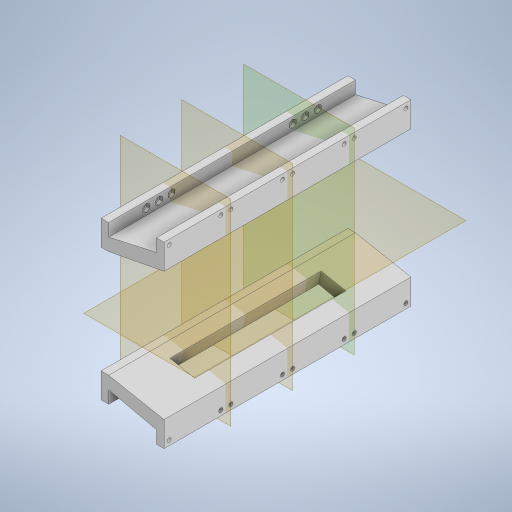
# Autodesk Inventor part: Antenna holder
Saved by Autodesk Inventor 2023.5 (Build 275446000, 446)
## iProperties
Created: 2025-10-16
Part Number: Antenna holder
Material: Generic
Document SubType Name: Modeling
Designer: Mikke
Density: 1 g/cm^3
Appearance: Default
Author: Mikke
Autodesk Inventor part; units mm, degrees
ref_plane "YZ Plane" through (0, 0, 0) normal (1, 0, 0) x (0, 1, 0)
ref_plane "XZ Plane" through (0, 0, 0) normal (0, 1, 0) x (-1, 0, 0)
ref_plane "XY Plane" through (0, 0, 0) normal (0, 0, 1) x (1, 0, 0)
sketch "Sketch4" plane through (0, 0, 0) normal (0, 0, 1) x (1, 0, 0)
  line L0 (-0.75, -71) -> (0.75, -71)
  line L1 (0.75, -71) -> (0.75, 71)
  line L2 (0.75, 71) -> (-0.75, 71)
  line L3 (-0.75, 71) -> (-0.75, -71)
  line L4 (-0.75, -71) -> (0.75, 71) construction
  line L5 (0.75, -71) -> (-0.75, 71) construction
  line L6 (-0.75, 71) -> (-6.75, 71)
  line L7 (-6.75, 71) -> (-6.75, 51)
  line L8 (-6.75, 51) -> (-0.75, 51)
  line L9 (-0.75, 51) -> (-0.75, 71)
  line L10 (-0.75, -71) -> (-6.75, -71)
  line L11 (-6.75, -71) -> (-6.75, -51)
  line L12 (-6.75, -51) -> (-0.75, -51)
  line L13 (-0.75, -51) -> (-0.75, -71)
  line L14 (-0.75, 0) -> (-50.75, 0)
  line L15 (-0.75, 0) -> (49.25, 0) construction
  line L16 (-0.75, 0) -> (-3.75, 0)
  line L17 (-6.75, -3) -> (-0.75, -3)
  line L18 (-0.75, -3) -> (-0.75, 3)
  line L19 (-0.75, 3) -> (-6.75, 3)
  line L20 (-6.75, 3) -> (-6.75, -3)
  line L21 (-6.75, -3) -> (-0.75, 3) construction
  line L22 (-0.75, -3) -> (-6.75, 3) construction
  line L23 (-6.75, 51) -> (-6.75, 61)
  line L24 (-6.75, -51) -> (-6.75, -61)
  line L25 (-50.75, 0) -> (-50.75, 62.5)
  line L26 (-50.75, 0) -> (-50.75, -62.5)
  line L27 (-50.75, 62.5) -> (-50.75, 52.5)
  line L28 (-50.75, -62.5) -> (-50.75, -62.5)
  line L29 (-50.75, 62.5) -> (-50.75, 57.5)
  line L30 (-50.75, -52.5) -> (-50.75, -57.5)
  line L31 (-50.75, 62.5) -> (-50.75, 42.5)
  line L32 (-50.75, 42.5) -> (-44.75, 42.5)
  line L33 (-44.75, 42.5) -> (-44.75, 62.5)
  line L34 (-44.75, 62.5) -> (-50.75, 62.5)
  line L35 (-50.75, 52.5) -> (-44.75, 52.5)
  line L36 (-44.75, 52.5) -> (-6.75, 61)
  line L37 (-50.75, -62.5) -> (-50.75, -42.5)
  line L38 (-50.75, -42.5) -> (-44.75, -42.5)
  line L39 (-44.75, -42.5) -> (-44.75, -62.5)
  line L40 (-44.75, -62.5) -> (-50.75, -62.5)
  line L41 (-50.75, -52.5) -> (-44.75, -52.5)
  line L42 (-44.75, -52.5) -> (-6.75, -61)
  line L43 (-44.75, -42.5) -> (-0.75, -51)
  line L44 (-44.75, 42.5) -> (-0.75, 51)
  point P0 (0, 0)
  point P1 (-0.75, -51)
  dimension "d22" = 1.5
  dimension "d23" = 142
  dimension "d24" = 6
  dimension "d25" = 20
  dimension "d26" = 6
  dimension "d27" = 20
  dimension "d28" = 50
  dimension "d29" = 180
  dimension "d36" = 6
  dimension "d37" = 6
  dimension "d38" = 10
  dimension "d39" = 10
  dimension "d45" = 62.5
  dimension "d46" = 62.5
  dimension "d47" = 10
  dimension "d55" = 115
  dimension "d56" = 20
  dimension "d57" = 6
  dimension "d58" = 20
  dimension "d59" = 6
  dimension "d60" = 20
  constraints: 90 end point, 10 midpoint, 9 perpendicular, 8 parallel, 6 horizontal, 5 point on line, 1 collinear, 1 vertical
  measures "d22" distance of L2.end L1.end
  measures "d23" distance of L1.end L0.end
  measures "d24" distance of L8.end L7.end
  measures "d25" distance of L7.end L6.end
  measures "d26" distance of L11.end L12.end
  measures "d27" distance of L10.end L11.end
  measures "d28" distance of L14.start L14.end
  measures "d29" angle of L14 L15
  measures "d36" distance of L19.end L18.end
  measures "d37" distance of L18.end L17.end
  measures "d38" distance of L7.end L23.end
  measures "d39" distance of L11.end L24.end
  measures "d45" distance of L14.end L25.end
  measures "d46" distance of L14.end L26.end
  measures "d47" distance of L25.end L27.end
  measures "d55" distance of L30.end L29.end
  measures "d56" distance of L25.end L31.end
  measures "d57" distance of L31.end L32.end
  measures "d58" distance of L28.start L37.end
  measures "d59" distance of L37.end L38.end
  measures "d60" distance of L38.end L39.end
extrude "Extrusion3" add sketch "Sketch4" along normal mid plane 196 contours L10 L11 L12 L3 | L12 L11 L42 L39 L43 | L39 L41 L26 L38 | L3 L8 L7 L6 | L39 L40 L26 L41 | L44 L33 L36 L7 L8 | L32 L25 L35 L33 | L35 L25 L34 L33
ref_plane "Work Plane4" through (0, 0, 0) normal (0, 0, 1) x (1, 0, 0)
ref_plane "Work Plane5" through (0, 0, -49) normal (0, 0, -1) x (-1, 0, 0)
ref_plane "Work Plane6" through (0, 0, 49) normal (0, 0, 1) x (1, 0, 0)
ref_plane "Work Plane7" through (-50.75, 0, 98) normal (0, 1, 0) x (1, 0, 0)
sketch "Sketch9" plane through (-6.75, 61, 98) normal (-1, 0, 0) x (0, 0, 1)
  line L0 (0, 10) -> (0, 0) projected
  line L1 (0, 10) -> (-24.5, 10)
  line L2 (0, 10) -> (-196, 10) projected
  line L3 (-24.5, 10) -> (-4, 10)
  line L4 (-24.5, 10) -> (-45, 10)
  line L5 (-45, 10) -> (-45, 6)
  line L6 (-45, 6) -> (-42.25, 6)
  line L7 (-4, 10) -> (-4, 6)
  line L8 (-4, 6) -> (-6.75, 6)
  line L9 (-6.75, 7.5877) -> (-4, 9.1754)
  line L10 (-4, 9.1754) -> (-1.25, 7.5877)
  line L11 (-1.25, 7.5877) -> (-1.25, 4.4123)
  line L12 (-1.25, 4.4123) -> (-4, 2.8246)
  line L13 (-4, 2.8246) -> (-6.75, 4.4123)
  line L14 (-6.75, 4.4123) -> (-6.75, 7.5877)
  line L15 (-42.25, 4.4123) -> (-45, 2.8246)
  line L16 (-45, 2.8246) -> (-47.75, 4.4123)
  line L17 (-47.75, 4.4123) -> (-47.75, 7.5877)
  line L18 (-47.75, 7.5877) -> (-45, 9.1754)
  line L19 (-45, 9.1754) -> (-42.25, 7.5877)
  line L20 (-42.25, 7.5877) -> (-42.25, 4.4123)
  point P0 (-98, -61)
  dimension "d88" = 24.5
  dimension "d89" = 20.5
  dimension "d90" = 20.5
  dimension "d91" = 4
  dimension "d92" = 2.75
  dimension "d93" = 4
  dimension "d94" = 2.75
  constraints: 38 end point, 3 point on line, 2 coincident, 2 horizontal, 2 midpoint, 2 perpendicular, 26 other
  measures "d88" distance of L0.start L1.end
  measures "d89" distance of L1.end L3.end
  measures "d90" distance of L1.end L4.end
  measures "d91" distance of L4.end L5.end
  measures "d92" distance of L5.end L6.end
  measures "d93" distance of L3.end L7.end
  measures "d94" distance of L7.end L8.end
extrude "Extrusion7" cut sketch "Sketch9" against normal blind 2.5
sketch "Sketch10" plane through (-4.25, 61, 98) normal (-1, 0, 0) x (0, 0, 1)
  line L0 (-4, 2.8246) -> (-6.75, 4.4123) projected
  line L1 (-4, 2.8246) -> (-4, 6.0001)
  circle A0 centre (-4, 6.0001) radius 1.55
  line L2 (-42.25, 4.4123) -> (-45, 2.8246) projected
  line L3 (-45, 2.8246) -> (-45, 6.0001)
  circle A1 centre (-45, 6.0001) radius 1.55
  point P0 (-98, -61)
  dimension "d97" = 3.1755
  dimension "d98" = 3.1
  dimension "d99" = 3.1755
  dimension "d100" = 3.1
  constraints: 4 end point, 2 centre point, 2 coincident, 2 vertical
  measures "d97" distance of L0.start L1.end
  measures "d98" diameter of A0
  measures "d99" distance of L2.end L3.end
  measures "d100" diameter of A1
extrude "Extrusion8" cut sketch "Sketch10" against normal blind 6
mirror "Mirror4" about plane through (0, 0, 49) normal (0, 0, 1) of "Extrusion7", "Extrusion8"
mirror "Mirror5" about plane through (0, 0, 0) normal (0, 0, 1) of "Extrusion7", "Extrusion8", "Mirror4"
mirror "Mirror6" about plane through (-50.75, 0, 98) normal (0, 1, 0) of "Extrusion7", "Extrusion8", "Mirror4", "Mirror5"
sketch "Sketch11" plane through (-44.75, 52.5, 98) normal (1, 0, 0) x (0, 0, -1)
  line L0 (196, 10) -> (0, 10) projected
  line L1 (98, 10) -> (49.925, 10)
  line L2 (196, 10) -> (0, 10) projected
  line L3 (98, 10) -> (146.075, 10)
  line L4 (49.925, 10) -> (49.925, 5)
  line L5 (49.925, 5) -> (52.675, 5)
  line L6 (146.075, 10) -> (146.075, 5)
  line L7 (146.075, 5) -> (143.325, 5)
  line L8 (49.925, 5) -> (39.925, 5)
  line L9 (39.925, 5) -> (42.675, 5)
  line L10 (39.925, 5) -> (29.925, 5)
  line L11 (29.925, 5) -> (32.675, 5)
  line L12 (146.075, 5) -> (156.075, 5)
  line L13 (156.075, 5) -> (153.325, 5)
  line L14 (156.075, 5) -> (166.075, 5)
  line L15 (166.075, 5) -> (163.325, 5)
  line L16 (143.325, 6.5877) -> (146.075, 8.1754)
  line L17 (146.075, 8.1754) -> (148.825, 6.5877)
  line L18 (148.825, 6.5877) -> (148.825, 3.4123)
  line L19 (148.825, 3.4123) -> (146.075, 1.8246)
  line L20 (146.075, 1.8246) -> (143.325, 3.4123)
  line L21 (143.325, 3.4123) -> (143.325, 6.5877)
  line L22 (153.325, 6.5877) -> (156.075, 8.1754)
  line L23 (156.075, 8.1754) -> (158.825, 6.5877)
  line L24 (158.825, 6.5877) -> (158.825, 3.4123)
  line L25 (158.825, 3.4123) -> (156.075, 1.8246)
  line L26 (156.075, 1.8246) -> (153.325, 3.4123)
  line L27 (153.325, 3.4123) -> (153.325, 6.5877)
  line L28 (163.325, 6.5877) -> (166.075, 8.1754)
  line L29 (166.075, 8.1754) -> (168.825, 6.5877)
  line L30 (168.825, 6.5877) -> (168.825, 3.4123)
  line L31 (168.825, 3.4123) -> (166.075, 1.8246)
  line L32 (166.075, 1.8246) -> (163.325, 3.4123)
  line L33 (163.325, 3.4123) -> (163.325, 6.5877)
  line L34 (52.675, 3.4123) -> (49.925, 1.8246)
  line L35 (49.925, 1.8246) -> (47.175, 3.4123)
  line L36 (47.175, 3.4123) -> (47.175, 6.5877)
  line L37 (47.175, 6.5877) -> (49.925, 8.1754)
  line L38 (49.925, 8.1754) -> (52.675, 6.5877)
  line L39 (52.675, 6.5877) -> (52.675, 3.4123)
  line L40 (42.675, 3.4123) -> (39.925, 1.8246)
  line L41 (39.925, 1.8246) -> (37.175, 3.4123)
  line L42 (37.175, 3.4123) -> (37.175, 6.5877)
  line L43 (37.175, 6.5877) -> (39.925, 8.1754)
  line L44 (39.925, 8.1754) -> (42.675, 6.5877)
  line L45 (42.675, 6.5877) -> (42.675, 3.4123)
  line L46 (32.675, 3.4123) -> (29.925, 1.8246)
  line L47 (29.925, 1.8246) -> (27.175, 3.4123)
  line L48 (27.175, 3.4123) -> (27.175, 6.5877)
  line L49 (27.175, 6.5877) -> (29.925, 8.1754)
  line L50 (29.925, 8.1754) -> (32.675, 6.5877)
  line L51 (32.675, 6.5877) -> (32.675, 3.4123)
  point P0 (98, -52.5)
  point P1 (98, -52.5)
  dimension "d103" = 48.075
  dimension "d104" = 48.075
  dimension "d105" = 5
  dimension "d106" = 2.75
  dimension "d107" = 5
  dimension "d108" = 2.75
  dimension "d109" = 10
  dimension "d110" = 2.75
  dimension "d111" = 10
  dimension "d112" = 2.75
  dimension "d113" = 10
  dimension "d114" = 2.75
  dimension "d115" = 10
  dimension "d116" = 2.75
  constraints: 100 end point, 7 coincident, 7 midpoint, 6 point on line, 4 horizontal, 3 perpendicular, 1 vertical, 78 other
  measures "d103" distance of L1.start L1.end
  measures "d104" distance of L1.start L3.end
  measures "d105" distance of L1.end L4.end
  measures "d106" distance of L4.end L5.end
  measures "d107" distance of L3.end L6.end
  measures "d108" distance of L6.end L7.end
  measures "d109" distance of L4.end L8.end
  measures "d110" distance of L8.end L9.end
  measures "d111" distance of L8.end L10.end
  measures "d112" distance of L10.end L11.end
  measures "d113" distance of L6.end L12.end
  measures "d114" distance of L12.end L13.end
  measures "d115" distance of L12.end L14.end
  measures "d116" distance of L14.end L15.end
extrude "Extrusion9" cut sketch "Sketch11" against normal blind 2.5
sketch "Sketch12" plane through (-47.25, 52.5, 98) normal (1, 0, 0) x (0, 0, -1)
  line L0 (166.075, 1.8246) -> (166.075, 5.0001)
  line L1 (166.075, 5.0001) -> (156.0758, 4.8772)
  line L2 (156.0758, 4.8772) -> (146.0765, 4.7544)
  circle A0 centre (146.0765, 4.7544) radius 1.55
  circle A1 centre (156.0758, 4.8772) radius 1.55
  circle A2 centre (166.075, 5.0001) radius 1.55
  line L3 (32.675, 3.4123) -> (29.925, 1.8246) projected
  line L4 (29.925, 1.8246) -> (29.925, 5.0001)
  line L5 (29.925, 5.0001) -> (39.925, 5.0001)
  line L6 (39.925, 5.0001) -> (49.925, 5.0001)
  circle A3 centre (29.925, 5.0001) radius 1.55
  circle A4 centre (39.925, 5.0001) radius 1.55
  circle A5 centre (49.925, 5.0001) radius 1.55
  point P0 (98, -52.5)
  dimension "d119" = 3.1755
  dimension "d120" = 10
  dimension "d121" = 10
  dimension "d122" = 180
  dimension "d123" = 3.1
  dimension "d124" = 3.1
  dimension "d125" = 3.1
  dimension "d126" = 3.1755
  dimension "d127" = 10
  dimension "d128" = 10
  dimension "d129" = 3.1
  dimension "d130" = 3.1
  dimension "d131" = 3.1
  constraints: 12 end point, 6 centre point, 6 coincident, 2 vertical, 1 collinear, 1 perpendicular, 1 point on line
  measures "d119" distance of L0.start L0.end
  measures "d120" distance of L0.end L1.end
  measures "d121" distance of L1.end L2.end
  measures "d122" angle of L2 L1
  measures "d123" diameter of A0
  measures "d124" diameter of A1
  measures "d125" diameter of A2
  measures "d126" distance of L3.end L4.end
  measures "d127" distance of L4.end L5.end
  measures "d128" distance of L5.end L6.end
  measures "d129" diameter of A3
  measures "d130" diameter of A4
  measures "d131" diameter of A5
extrude "Extrusion10" cut sketch "Sketch12" against normal blind 6
mirror "Mirror7" about plane through (-50.75, 0, 98) normal (0, 1, 0) of "Extrusion9", "Extrusion10"
sketch "Sketch15" plane through (-44.75, -42.5, 98) normal (0.1897, 0.9818, 0) x (0.9818, -0.1897, 0)
  line L0 (35.8765, 98) -> (20.8765, 98)
  line L1 (0, 196) -> (0, 0) projected
  line L2 (35.8765, 98) -> (50.8765, 98) construction
  line L3 (30.8765, 38) -> (10.8765, 38)
  line L4 (10.8765, 38) -> (10.8765, 158)
  line L5 (10.8765, 158) -> (30.8765, 158)
  line L6 (30.8765, 158) -> (30.8765, 38)
  line L7 (30.8765, 38) -> (10.8765, 158) construction
  line L8 (10.8765, 38) -> (30.8765, 158) construction
  dimension "d142" = 15
  dimension "d143" = 180
  dimension "d144" = 20
  dimension "d145" = 120
  constraints: 16 end point, 2 horizontal, 2 midpoint, 2 parallel, 2 perpendicular, 1 collinear
  measures "d142" distance of L0.start L0.end
  measures "d143" angle of L0 L2
  measures "d144" distance of L4.end L5.end
  measures "d145" distance of L3.end L4.end
extrude "Extrusion12" cut sketch "Sketch15" against normal blind 14
body "Solid2"
